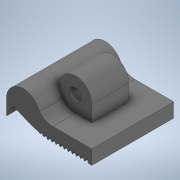
# Autodesk Inventor part: Nail
Saved by Autodesk Inventor 2020 (Build 240168000, 168)
## iProperties
Created: 2019-10-18
Part Number: Nail
Material: Generic
Document SubType Name: Modeling
Designer: ayad493
Density: 1 g/cm^3
Appearance: Gray
Author: ayad493
Autodesk Inventor part; units mm, degrees
ref_plane "YZ Plane" through (0, 0, 0) normal (1, 0, 0) x (0, 1, 0)
ref_plane "XZ Plane" through (0, 0, 0) normal (0, 1, 0) x (-1, 0, 0)
ref_plane "XY Plane" through (0, 0, 0) normal (0, 0, 1) x (1, 0, 0)
sketch "Sketch23" plane through (0, 0, 0) normal (0, 0, 1) x (1, 0, 0)
  arc A0 (4, 0) -> (0, -4) centre (0, 0) ccw
  line L0 (-4, 0) -> (4, 0)
  line L1 (4, 0) -> (4, -4.25)
  line L2 (0, -4) -> (-3.2578, -4)
  line L3 (-4, -1.4182) -> (-4, 0)
  line L4 (10.5, -4.25) -> (10.5, -7.75)
  line L5 (10.5, -7.75) -> (-4.5, -7.75)
  line L6 (-7.75, -4.25) -> (-7.25, -4.25)
  line L7 (-3.2578, -4) -> (0, -4)
  line L8 (4, -4.25) -> (10.5, -4.25)
  line L9 (-7.25, -4.25) -> (-7.25, -3.75)
  arc A1 (-3.2578, -4) -> (-11.25, -3.75) centre (-7.25, -3.75) ccw
  line L10 (-11.25, -3.75) -> (-11.25, -7.75)
  line L11 (-7.25, -7.75) -> (-11.25, -7.75)
  line L12 (-7.25, -7.75) -> (-4.5, -7.75)
  dimension "d140" = 8
  dimension "d141" = 15
  dimension "d142" = 3.5
  dimension "d143" = 4.25
  dimension "d166" = 0.5
  dimension "d167" = 8
  constraints: 26 end point, 6 point on circle, 4 horizontal, 4 parallel, 3 perpendicular, 3 tangent, 2 centre point, 2 coincident, 1 vertical
  measures "d140" diameter of A0
  measures "d141" distance of L4.end L5.end
  measures "d142" distance of L4.start L4.end
  measures "d143" distance of L0.end L1.end
  measures "d166" distance of L6.end L9.end
  measures "d167" diameter of A1
extrude "Extrusion25" add sketch "Sketch23" along normal blind 20 contours L0 A0 | L1 L8 L4 L5 L12 L11 L10 A1 L2 A0 L0
sketch "Sketch30" plane through (0, 0, 20) normal (0, 0, 1) x (1, 0, 0)
  circle A0 centre (0, 0) radius 1.5
  dimension "d168" = 3
  constraints: 1 centre point, 1 coincident
  measures "d168" diameter of A0
extrude "Extrusion30" cut sketch "Sketch30" against normal through all
sketch "Sketch31" plane through (0, 0, 20) normal (0, 0, 1) x (1, 0, 0)
  line L0 (0, -4) -> (10.5, -4)
  line L1 (10.5, -7.75) -> (10.5, -4.25) projected
  line L2 (10.5, -4) -> (10.5, -7.75)
  line L3 (-11.25, -7.75) -> (10.5, -7.75) projected
  line L4 (0, -4) -> (10.5, -4)
  line L5 (10.5, -4) -> (10.5, -7.75)
  line L6 (10.5, -7.75) -> (0, -7.75)
  line L7 (0, -7.75) -> (0, -4)
  point P0 (0, 0)
  point P1 (0, -7.75)
  constraints: 12 end point, 2 horizontal, 2 parallel, 1 collinear, 1 perpendicular
extrude "Extrusion31" add sketch "Sketch31" against normal up to surface (20 mm away)
sketch "Sketch32" plane through (0, 0, 20) normal (0, 0, 1) x (1, 0, 0)
  circle A0 centre (0, 0) radius 4
  line L0 (4, -4) -> (10.5, -4) projected
  line L1 (0, 0) -> (4, 0)
  line L2 (4, 0) -> (4, -4)
  line L3 (4, -4) -> (0, -4)
  line L4 (0, -4) -> (0, 0)
  circle A1 centre (0, 0) radius 1.5
  constraints: 8 end point, 2 centre point, 2 coincident, 2 parallel, 1 horizontal, 1 perpendicular
extrude "Extrusion32" cut sketch "Sketch32" against normal blind 5.5 contours L1 A1 L4 A0 | L2 L3 A0 | A0 L4 A1 L1
sketch "Sketch33" plane through (0, 0, 0) normal (0, 0, -1) x (-1, 0, 0)
  circle A0 centre (0, 0) radius 4
  circle A1 centre (0, 0) radius 1.5
  line L0 (-10.5, -4) -> (3.2578, -4) projected
  line L1 (0, 0) -> (-4, 0)
  line L2 (-4, 0) -> (-4, -4)
  line L3 (-4, -4) -> (0, -4)
  line L4 (0, -4) -> (0, 0)
  point P0 (0, -4)
  constraints: 8 end point, 2 centre point, 2 coincident, 2 parallel, 1 horizontal, 1 perpendicular, 1 point on line
extrude "Extrusion33" cut sketch "Sketch33" against normal blind 5.5 contours A0 L4 A1 L1 | L1 A1 L4 A0 | A0 L0 L2
fillet "Fillet3" radius 4.25 1 edges at (-3.2578, -4, 10)
sketch "Sketch34" plane through (0, 0, 20) normal (0, 0, 1) x (1, 0, 0)
  arc A0 (-3.7516, -1.8106) -> (-11.25, -3.75) centre (-7.25, -3.75) ccw projected
  circle A1 centre (-7.25, -3.75) radius 4.1624
  arc A2 (4, 0) -> (0, -4) centre (0, 0) ccw projected
  line L0 (-11.25, -7.75) -> (10.5, -7.75) projected
  line L1 (-8.4014, -7.75) -> (-6.0986, -7.75)
  line L2 (-11.25, -3.75) -> (-11.25, -7.75) projected
  arc A3 (-11.4124, -3.75) -> (-11.25, -7.75) centre (8.552, -4.9427) ccw
  line L3 (-11.25, -7.75) -> (-6.0986, -7.75)
  dimension "d185" = 20
  constraints: 5 point on circle, 4 end point, 2 centre point, 2 point on line, 1 coincident, 1 perpendicular, 1 tangent
  measures "d185" radius of A3
extrude "Extrusion36" add sketch "Sketch34" against normal up to surface (20 mm away) contours L0 L2 A1 | A1 L0 | L2 A3 A1 picked at (-6.2004, -2.965)
sketch "Sketch35" plane through (0, 0, 20) normal (0, 0, 1) x (1, 0, 0)
  line L0 (10.5, -7.75) -> (10.5, -4) projected
  arc A0 (-11.4124, -3.75) -> (-11.25, -7.75) centre (8.552, -4.9427) ccw projected
  line L1 (10.5, -7.75) -> (-11.2838, -7.75)
  line L2 (-11.2838, -7.75) -> (-11.2838, -7.5)
  line L3 (-11.2838, -7.5) -> (10.5, -7.5)
  line L4 (10.5, -7.5) -> (10.5, -7.75)
  point P0 (0, 0)
  point P1 (10.5, -7.5)
  point P2 (-11.25, -7.75)
  dimension "d188" = 0.25
  constraints: 8 end point, 2 parallel, 1 horizontal, 1 perpendicular, 1 point on circle
  measures "d188" distance of L1.end L2.end
extrude "Extrusion37" cut sketch "Sketch35" against normal through all contours L1 A0 L3 L0
sketch "Sketch36" plane through (0, 0, 20) normal (0, 0, 1) x (1, 0, 0)
  line L0 (-11.2838, -7.5) -> (10.5, -7.5) projected
  line L1 (10.5, -4) -> (-0.0346, -4) projected
  line L2 (10.5, -7.5) -> (9.5, -7.5)
  line L3 (9.5, -7.5) -> (9.5, -4)
  line L4 (9.5, -4) -> (10.5, -4)
  line L5 (10.5, -4) -> (10.5, -7.5)
  point P0 (0, 0)
  dimension "d191" = 1
  constraints: 8 end point, 2 parallel, 1 horizontal, 1 perpendicular, 1 point on line
  measures "d191" distance of L3.end L4.end
extrude "Extrusion38" cut sketch "Sketch36" against normal through all
sketch "Sketch38" plane through (0, 0, 0) normal (0, 0, -1) x (-1, 0, 0)
  arc A0 (11.2838, -7.5) -> (11.4124, -3.75) centre (-8.552, -4.9427) ccw projected
  line L0 (11.2838, -7.5) -> (10.7838, -6.634)
  line L1 (11.2838, -7.5) -> (12.2838, -7.5) construction
  line L2 (10.7838, -6.634) -> (10.2838, -7.5)
  line L3 (-9.5, -7.5) -> (11.2838, -7.5) projected
  line L4 (10.2838, -7.5) -> (9.7838, -6.634)
  line L5 (9.7838, -6.634) -> (9.2838, -7.5)
  line L6 (9.2838, -7.5) -> (8.7838, -6.634)
  line L7 (8.7838, -6.634) -> (8.2838, -7.5)
  line L8 (8.2838, -7.5) -> (7.7838, -6.634)
  line L9 (7.7838, -6.634) -> (7.2838, -7.5)
  line L10 (7.2838, -7.5) -> (6.7838, -6.634)
  line L11 (6.7838, -6.634) -> (6.2838, -7.5)
  line L12 (6.2838, -7.5) -> (5.7838, -6.634)
  line L13 (5.7838, -6.634) -> (5.2838, -7.5)
  line L14 (5.2838, -7.5) -> (4.7838, -6.634)
  line L15 (4.7838, -6.634) -> (4.2838, -7.5)
  line L16 (4.2838, -7.5) -> (3.7838, -6.634)
  line L17 (3.7838, -6.634) -> (3.2838, -7.5)
  line L18 (3.2838, -7.5) -> (2.7838, -6.634)
  line L19 (2.7838, -6.634) -> (2.2838, -7.5)
  line L20 (2.2838, -7.5) -> (1.7838, -6.634)
  line L21 (1.7838, -6.634) -> (1.2838, -7.5)
  line L22 (1.2838, -7.5) -> (0.7838, -6.634)
  line L23 (0.7838, -6.634) -> (0.2838, -7.5)
  line L24 (0.2838, -7.5) -> (-0.2162, -6.634)
  line L25 (-0.2162, -6.634) -> (-0.7162, -7.5)
  line L26 (-0.7162, -7.5) -> (-1.2162, -6.634)
  line L27 (-1.2162, -6.634) -> (-1.7162, -7.5)
  line L28 (-1.7162, -7.5) -> (-2.2162, -6.634)
  line L29 (-2.2162, -6.634) -> (-2.7162, -7.5)
  line L30 (-2.7162, -7.5) -> (-3.2162, -6.634)
  line L31 (-3.2162, -6.634) -> (-3.7162, -7.5)
  line L32 (-3.7162, -7.5) -> (-4.2162, -6.634)
  line L33 (-4.2162, -6.634) -> (-4.7162, -7.5)
  line L34 (-4.7162, -7.5) -> (-5.2162, -6.634)
  line L35 (-5.2162, -6.634) -> (-5.7162, -7.5)
  line L36 (-5.7162, -7.5) -> (-6.2162, -6.634)
  line L37 (-6.2162, -6.634) -> (-6.7162, -7.5)
  line L38 (-6.7162, -7.5) -> (-7.2162, -6.634)
  line L39 (-7.2162, -6.634) -> (-7.7162, -7.5)
  line L40 (-7.7162, -7.5) -> (-8.2162, -6.634)
  line L41 (-8.2162, -6.634) -> (-8.7162, -7.5)
  line L42 (11.2838, -7.5) -> (-8.7162, -7.5)
  point P0 (0, 0)
  dimension "d205" = 1
  dimension "d206" = 120
  dimension "d209" = 1
  constraints: 84 end point, 57 horizontal alignment, 38 parallel, 2 horizontal, 1 equal length, 2 other
  measures "d205" distance of L0.start L0.end
  measures "d206" angle of L1 L0
  measures "d209" distance of L0.start L4.start
extrude "Extrusion40" cut sketch "Sketch38" against normal through all
sketch "Sketch39" plane through (0, 0, 20) normal (0, 0, 1) x (1, 0, 0)
  arc A0 (-11.4124, -3.75) -> (-11.2838, -7.5) centre (8.552, -4.9427) ccw projected
  line L0 (-11.4124, -3.75) -> (-11.4124, -7.5)
  line L1 (-10.7838, -6.634) -> (-11.2838, -7.5) projected
  line L2 (-11.4124, -7.5) -> (-10.7838, -6.634)
  line L3 (-10.7838, -6.634) -> (-11.4124, -3.75)
  point P0 (0, 0)
  point P1 (-11.4124, -6.1353)
  point P2 (-11.3027, -7.3489)
  constraints: 6 end point, 1 vertical
extrude "Extrusion41" add sketch "Sketch39" against normal up to surface (20 mm away) contours L3 L2 A0 L0 | A0 L2 L0
sketch "Sketch40" plane through (0, 0, 20) normal (0, 0, 1) x (1, 0, 0)
  line L0 (-11.4124, -6.1353) -> (-11.4124, -7.5) projected
  line L1 (-11.4124, -7.5) -> (-11.4124, 0)
  line L2 (-11.4124, -7.5) -> (-3.9124, -7.5) construction
  line L3 (-11.4124, 0) -> (-12.4534, 0)
  line L4 (-12.4534, 0) -> (-12.4534, -7.5)
  line L5 (-12.4534, -7.5) -> (-11.4124, -7.5)
  line L6 (-11.4124, -7.5) -> (-10.7811, -6.63)
  line L7 (-11.4124, -7.5) -> (-10.3375, -7.5) construction
  line L8 (-10.7811, -6.63) -> (-10.7811, -7.5)
  line L9 (-11.4124, -7.5) -> (-10.7811, -7.5)
  point P0 (0, 0)
  dimension "d218" = 90
  dimension "d219" = 54.03
  constraints: 18 end point, 4 perpendicular, 2 equal length, 2 horizontal, 1 collinear, 1 point on line
  measures "d218" angle of L2 L1
  measures "d219" angle of L7 L6
extrude "Extrusion42" cut sketch "Sketch40" against normal through all
sketch "Sketch41" plane through (0, 0, 20) normal (0, 0, 1) x (1, 0, 0)
  line L0 (-11.4124, -7.5) -> (-11.4124, -3.75) projected
  line L1 (-11.4124, -7.5) -> (-10.2377, -5.8814)
  line L2 (-11.4124, -7.5) -> (-9.4124, -7.5) construction
  line L3 (-9.7838, -6.634) -> (-10.2838, -7.5) projected
  line L4 (-10.2377, -5.8814) -> (-10.2838, -7.5)
  line L5 (-10.2838, -7.5) -> (-10.7839, -6.6339)
  line L6 (-10.2838, -7.5) -> (-10.7811, -6.6388) projected
  point P0 (0, 0)
  dimension "d222" = 2
  dimension "d223" = 54.03
  constraints: 8 end point, 1 collinear, 1 equal length, 1 horizontal, 1 point on line
  measures "d222" distance of L0.start L1.end
  measures "d223" angle of L2 L1
extrude "Extrusion43" cut sketch "Sketch41" against normal through all
sketch "Sketch42" plane through (0, 0, 20) normal (0, 0, 1) x (1, 0, 0)
  line L0 (-11.3027, -7.3489) -> (-11.4124, -7.5) projected
  line L1 (-11.4124, -7.5) -> (-9.6624, -4.4689)
  line L2 (-11.4124, -7.5) -> (-7.9124, -7.5) construction
  line L3 (-9.2838, -7.5) -> (-8.7838, -6.634) projected
  line L4 (-9.6624, -4.4689) -> (-9.2838, -7.5)
  line L5 (-11.4124, -7.5) -> (-11.4124, -3.75) projected
  line L6 (-9.2838, -7.5) -> (-11.4124, -7.5)
  arc A0 (-9.6624, -4.4689) -> (-1.2838, -7.5) centre (6.3367, 26.6603) ccw
  line L7 (-9.2838, -7.5) -> (-9.7838, -6.634) projected
  line L8 (-9.2838, -7.5) -> (-1.2838, -7.5)
  point P0 (0, 0)
  point P1 (-1.2838, -7.5)
  dimension "d226" = 3.5
  dimension "d227" = 60
  dimension "d230" = 35
  constraints: 10 end point, 2 point on circle, 1 centre point, 1 equal length, 1 horizontal, 1 perpendicular, 1 point on line
  measures "d226" distance of L0.end L1.end
  measures "d227" angle of L2 L1
  measures "d230" radius of A0
extrude "Extrusion44" cut sketch "Sketch42" against normal through all
body "Solid3"
